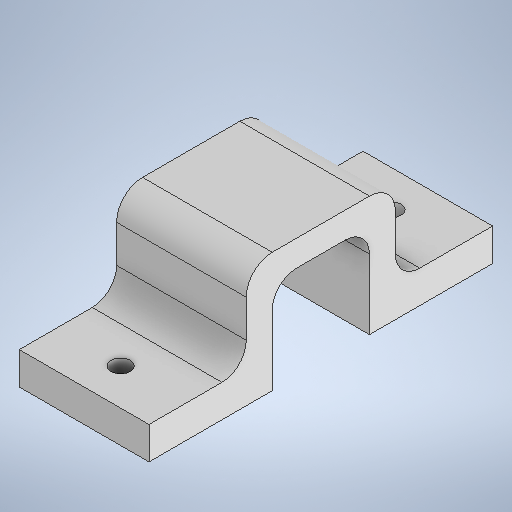
# Autodesk Inventor part: TubeHolderV1
Saved by Autodesk Inventor 2025.1 (Build 291241020, 241B)
## iProperties
Created: 2025-05-04
Part Number: TubeHolderV1
Material: Generic
Document SubType Name: Modeling
Designer: dpseu
Density: 1 g/cm^3
Appearance: Default
Author: dpseu
Autodesk Inventor part; units mm, degrees
ref_plane "YZ Plane" through (0, 0, 0) normal (1, 0, 0) x (0, 1, 0)
ref_plane "XZ Plane" through (0, 0, 0) normal (0, 1, 0) x (-1, 0, 0)
ref_plane "XY Plane" through (0, 0, 0) normal (0, 0, 1) x (1, 0, 0)
sketch "Sketch1" plane through (0, 0, 0) normal (0, 1, 0) x (-1, 0, 0)
  line L0 (0, 0) -> (18.415, 0)
  line L1 (18.415, 0) -> (18.415, -19.05)
  line L2 (18.415, -19.05) -> (0, -19.05)
  line L3 (0, 0) -> (0, 5.08)
  line L4 (6.35, 5.08) -> (23.495, 5.08)
  line L5 (23.495, 5.08) -> (23.495, -24.13)
  line L6 (23.495, -24.13) -> (6.35, -24.13)
  line L7 (0, -23.495) -> (0, -19.05)
  line L8 (0, 5.08) -> (0, 24.13)
  line L9 (0, 24.13) -> (6.35, 24.13)
  line L10 (6.35, 24.13) -> (6.35, 5.08)
  line L11 (0, -23.495) -> (0, -43.18)
  line L12 (0, -43.18) -> (6.35, -43.18)
  line L13 (6.35, -43.18) -> (6.35, -24.13)
  dimension "d2" = 18.415
  dimension "d3" = 19.05
  dimension "d4" = 18.415
  dimension "d5" = 5.08
  dimension "d6" = 5.08
  dimension "d7" = 5.08
  dimension "d8" = 6.35
  dimension "d9" = 6.35
  dimension "d10" = 24.13
  dimension "d11" = 24.13
  constraints: 28 end point, 8 perpendicular, 3 vertical, 1 horizontal, 1 parallel, 1 point on line
  measures "d2" distance of L0.start L0.end
  measures "d3" distance of L0.end L1.end
  measures "d4" distance of L1.end L2.end
  measures "d5" distance between parallel lines of L0 L4
  measures "d6" distance between parallel lines of L5 L1
  measures "d7" distance between parallel lines of L6 L2
  measures "d8" distance between parallel lines of L10 L8
  measures "d9" distance between parallel lines of L13 L11
  measures "d10" distance between parallel lines of L9 L0
  measures "d11" distance between parallel lines of L12 L2
extrude "Extrusion1" add sketch "Sketch1" along normal blind 25.4
fillet "Fillet1" radius 4.7625 1 edges at (-18.415, 12.7, 0)
fillet "Fillet2" radius 4.7625 1 edges at (-18.415, 12.7, -19.05)
fillet "Fillet3" radius 4.7625 1 edges at (-6.35, 12.7, 5.08)
fillet "Fillet4" radius 4.7625 1 edges at (-6.35, 12.7, -24.13)
fillet "Fillet5" radius 5.08 2 edges at (-23.495, 12.7, 5.08) (-23.495, 12.7, -24.13)
sketch "Sketch3" plane through (-6.35, 0, 24.13) normal (-1, 0, 0) x (0, 0, 1)
  circle A0 centre (-7.1501, 12.7) radius 1.905
  line L0 (-14.2875, 0) -> (0, 0) projected
  line L1 (0, 0) -> (0, 25.4) projected
  point P0 (-24.13, 0)
  dimension "d31" = 3.81
  dimension "d32" = 12.7
  dimension "d33" = 7.1501
  constraints: 1 centre point
  measures "d31" diameter of A0
  measures "d32" distance from line of L0 A0.centre
  measures "d33" distance from line of L1 A0.centre
extrude "Extrusion2" cut sketch "Sketch3" against normal up to surface (6.35 mm away)
sketch "Sketch4" plane through (-6.35, 0, -43.18) normal (-1, 0, 0) x (0, 0, 1)
  circle A0 centre (7.1501, 12.7) radius 1.905
  line L0 (0, 0) -> (14.2875, 0) projected
  line L1 (0, 0) -> (0, 25.4) projected
  point P0 (43.18, 0)
  dimension "d36" = 3.81
  dimension "d37" = 12.7
  dimension "d38" = 7.1501
  constraints: 1 centre point
  measures "d36" diameter of A0
  measures "d37" distance from line of L0 A0.centre
  measures "d38" distance from line of L1 A0.centre
extrude "Extrusion3" cut sketch "Sketch4" against normal up to surface (6.35 mm away)
body "Solid1"
